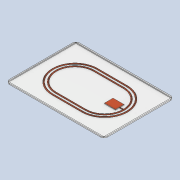
# Autodesk Inventor part: Playing Card RFID Inside
Saved by Autodesk Inventor 2021 (Build 250183000, 183)
## iProperties
Created: 2021-03-18
Part Number: Playing Card RFID Inside
Material: Generic
Document SubType Name: Modeling
Designer: calst
Density: 1 g/cm^3
Appearance: Smooth - White
Author: calst
Autodesk Inventor part; units mm, degrees
ref_plane "YZ Plane" through (0, 0, 0) normal (1, 0, 0) x (0, 1, 0)
ref_plane "XZ Plane" through (0, 0, 0) normal (0, 1, 0) x (-1, 0, 0)
sketch "Sketch1" plane through (0, 0, 0) normal (0, 1, 0) x (-1, 0, 0)
  line L0 (0, 0) -> (88.9, 0)
  line L1 (88.9, 0) -> (88.9, -63.5)
  line L2 (88.9, -63.5) -> (0, -63.5)
  line L3 (0, -63.5) -> (0, 0)
  dimension "d0" = 63.5
  dimension "d1" = 88.9
  constraints: 8 end point, 2 parallel, 1 horizontal, 1 perpendicular
  measures "d0" distance of L0.end L1.end
  measures "d1" distance of L0.start L0.end
extrude "Extrusion1" add sketch "Sketch1" along normal blind 1
sketch "Sketch2" plane through (0, 1, 0) normal (0, 1, 0) x (1, 0, 0)
  line L0 (-87.9, 62.3439) -> (-1, 62.3439)
  line L1 (-1, 62.3439) -> (-1, 0.8798)
  line L2 (-1, 0.8798) -> (-87.9, 0.8798)
  line L3 (-87.9, 0.8798) -> (-87.9, 62.3439)
  point P0 (0, 0)
  constraints: 8 end point, 2 parallel, 1 horizontal, 1 perpendicular
extrude "Extrusion2" cut sketch "Sketch2" against normal blind 0.8
sketch "Sketch3" plane through (0, 0.2, 0) normal (0, 1, 0) x (1, 0, 0)
  line L0 (-57.9, 31.6119) -> (-31, 31.6119) construction
  line L1 (-57.9, 10.8798) -> (-31, 10.8798)
  line L2 (-31, 52.3439) -> (-57.9, 52.3439)
  arc A0 (-57.9, 52.3439) -> (-57.9, 10.8798) centre (-57.9, 31.6119) ccw
  arc A1 (-31, 10.8798) -> (-31, 52.3439) centre (-31, 31.6119) ccw
  line L3 (-87.9, 62.3439) -> (-1, 62.3439) projected
  line L4 (-1, 0.8798) -> (-87.9, 0.8798) projected
  line L5 (-87.9, 0.8798) -> (-87.9, 62.3439) projected
  line L6 (-1, 62.3439) -> (-1, 0.8798) projected
  line L7 (-57.9, 31.6119) -> (-31, 31.6119) construction
  line L8 (-57.9, 12.0677) -> (-31, 12.0677)
  line L9 (-31, 51.1561) -> (-57.9, 51.1561)
  arc A2 (-57.9, 51.1561) -> (-57.9, 12.0677) centre (-57.9, 31.6119) ccw
  arc A3 (-31, 12.0677) -> (-31, 51.1561) centre (-31, 31.6119) ccw
  line L10 (-57.9, 31.6119) -> (-31, 31.6119) construction
  line L11 (-57.9, 13.7692) -> (-31, 13.7692)
  line L12 (-31, 49.4545) -> (-57.9, 49.4545)
  arc A4 (-57.9, 49.4545) -> (-57.9, 13.7692) centre (-57.9, 31.6119) ccw
  arc A5 (-31, 13.7692) -> (-31, 49.4545) centre (-31, 31.6119) ccw
  line L13 (-57.9, 31.6119) -> (-31, 31.6119) construction
  line L14 (-57.9, 14.9514) -> (-31, 14.9514)
  line L15 (-31, 48.2724) -> (-57.9, 48.2724)
  arc A6 (-57.9, 48.2724) -> (-57.9, 14.9514) centre (-57.9, 31.6119) ccw
  line L16 (-6.3537, 31.9899) -> (-6.3537, 31.6119)
  line L17 (-6.3537, 31.2338) -> (-22.3253, 31.9899) construction
  line L18 (-22.3253, 31.2338) -> (-6.3537, 31.9899) construction
  arc A7 (-31, 14.9514) -> (-14.3438, 31.2338) centre (-31, 31.6119) ccw
  arc A8 (-14.3438, 31.9899) -> (-31, 48.2724) centre (-31, 31.6119) ccw
  line L19 (-27.3253, 27.6746) -> (-17.3253, 27.6746)
  line L20 (-17.3253, 27.6746) -> (-17.3253, 35.5491)
  line L21 (-17.3253, 35.5491) -> (-27.3253, 35.5491)
  line L22 (-27.3253, 35.5491) -> (-27.3253, 27.6746)
  line L23 (-27.3253, 27.6746) -> (-17.3253, 35.5491) construction
  line L24 (-17.3253, 27.6746) -> (-27.3253, 35.5491) construction
  line L25 (-17.3253, 31.9899) -> (-14.3438, 31.9899)
  line L26 (-14.3438, 31.2338) -> (-17.3253, 31.2338)
  point P0 (0, 0)
  point P1 (-44.45, 31.6119)
  point P2 (-44.45, 31.6119)
  point P3 (-44.45, 31.6119)
  point P4 (-44.45, 31.6119)
  dimension "d8" = 10
  dimension "d9" = 10
  dimension "d10" = 30
  dimension "d11" = 30
  dimension "d12" = 10
  constraints: 54 end point, 18 point on circle, 16 tangent, 10 equal length, 9 centre point, 4 midpoint, 3 horizontal, 3 point on line, 1 perpendicular
  measures "d8" distance between parallel lines of L3 L2
  measures "d9" distance between parallel lines of L4 L1
  measures "d10" distance from line of L5 L0.start
  measures "d11" distance from line of L6 L0.end
  measures "d12" distance of L21.end L20.end
extrude "Extrusion3" add sketch "Sketch3" along normal blind 0.6 contours A0 L2 A1 L1 | A4 L12 A5 L11 | L20 L19 L22 L21
fillet "Fillet3" radius 0.5 12 edges at (-44.45, 0.8, -10.8798) (-10.268, 0.8, -31.6119) (-44.45, 0.8, -52.3439) (-78.632, 0.8, -31.6119) (-44.45, 0.8, -51.1561) (-11.4558, 0.8, -31.6119) (-44.45, 0.8, -12.0677) (-77.4442, 0.8, -31.6119) (-44.45, 0.8, -13.7692) (-13.1574, 0.8, -31.6119) (-44.45, 0.8, -49.4545) (-75.7426, 0.8, -31.6119)
fillet "Fillet4" radius 0.5 5 edges at (-44.45, 0.8, -14.9514) (-74.5605, 0.8, -31.6119) (-44.45, 0.8, -48.2724) (-19.3537, 0.8, -43.5255) (-19.3537, 0.8, -19.6982)
fillet "Fillet5" radius 0.3 4 edges at (-14.0937, 0.8, -31.2338) (-15.8345, 0.8, -31.2338) (-14.0937, 0.8, -31.9899) (-15.8345, 0.8, -31.9899)
fillet "Fillet6" radius 3 1 edges at (0, 0.5, -63.5)
fillet "Fillet7" radius 3 3 edges at (-88.9, 0.5, -63.5) (-88.9, 0.5, 0) (0, 0.5, 0)
ref_plane "Work Plane2" through (0, -5, 0) normal (0, -1, 0) x (1, 0, 0)
body "Solid1"
